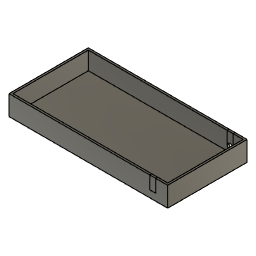
Enclosure_alpha v2 (Autodesk Fusion 360 design; units mm, degrees)
Autodesk Fusion 360 part; units mm, degrees
sketch "Sketch1" plane through (0, 0, 0) normal (0, 0, 1) x (1, 0, 0)
  line L0 (0, 0) -> (160, 0)
  line L1 (160, 0) -> (160, 80)
  line L2 (160, 80) -> (0, 80)
  line L3 (0, 80) -> (0, 0)
  line L4 (2, 2) -> (158, 2)
  line L5 (158, 2) -> (158, 78)
  line L6 (158, 78) -> (2, 78)
  line L7 (2, 78) -> (2, 2)
  constraint horizontal L0
  constraint vertical L1
  constraint horizontal L2
  constraint vertical L3
  constraint coincident L0.start L3.end
  constraint horizontal L4
  constraint vertical L5
  constraint horizontal L6
  constraint vertical L7
extrude "Extrude1" add sketch "Sketch1" along normal blind 20 makes body 1
sketch "Sketch2" plane through (0, 0, 0) normal (0, 0, 1) x (1, 0, 0)
  line L0 (2, 2) -> (158, 2)
  line L1 (158, 2) -> (158, 78)
  line L2 (158, 78) -> (2, 78)
  line L3 (2, 78) -> (2, 2)
  constraint horizontal L0
  constraint vertical L1
  constraint horizontal L2
  constraint vertical L3
extrude "Extrude2" add sketch "Sketch2" along normal blind 2 bodies 1
sketch "Sketch3" plane through (0, 80, 0) normal (0, 1, 0) x (-1, 0, 0)
  line L0 (-160, 0) -> (0, 0)
  line L1 (0, 0) -> (0, 20)
  line L2 (0, 20) -> (-160, 20)
  line L3 (-160, 20) -> (-160, 0)
  circle A0 centre (-144.9737, 7) radius 2.8021
  line L4 (-142.1716, 7) -> (-142.1716, 20)
  line L5 (-147.7758, 7) -> (-147.7758, 20)
  line L6 (-147.7758, 20) -> (-142.1716, 20)
  constraint coincident A0 L4.start
  constraint coincident L2 L4.end
  constraint tangent A0 L4
  constraint perpendicular L2 L4
  constraint coincident A0 L5.start
  constraint coincident L2 L5.end
  constraint tangent A0 L5
  constraint perpendicular L2 L5
hole "Hole1" at (144.9737, 80, 7) direction (0, -1, 0) diameter 6 depth 9 tip angle 180 bodies 1
sketch "Sketch4" plane through (0, 80, 0) normal (0, 1, 0) x (-1, 0, 0)
  circle A0 centre (-144.9737, 7) radius 3
  line L0 (-160, 0) -> (0, 0)
  line L1 (0, 0) -> (0, 20)
  line L2 (0, 20) -> (-160, 20)
  line L3 (-160, 20) -> (-160, 0)
  line L4 (-147.9737, 7.0059) -> (-141.9737, 7.0059)
  line L5 (-141.9737, 7.0059) -> (-141.999, 20)
  line L6 (-147.9737, 7.0059) -> (-147.9483, 20)
  line L7 (-147.9483, 20) -> (-141.999, 20)
  constraint coincident A0 L4.start
  constraint coincident A0 L4.end
  constraint horizontal L4
  constraint coincident L2 L5.end
  constraint tangent A0 L5
  constraint coincident L2 L6.end
  constraint tangent A0 L6
split "Split1" by curves path "Sketch4" along L7 L6 L4 L5 bodies 1 makes body 2 at (144.9737, 80, 16.6667) makes body 3 at (53.3333, 53.3333, 0)
